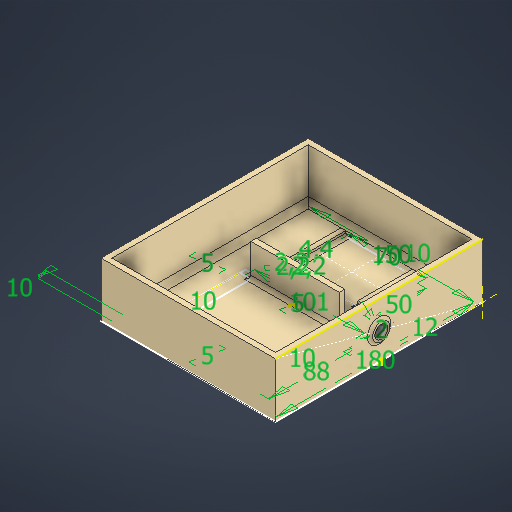
# Autodesk Inventor part: CaseBitDog
Saved by Autodesk Inventor 2027 (Build 310192000, 192)
## iProperties
Created: 2026-10-02
Part Number: CaseBitDog
Material: Genérico
Document SubType Name: Modeling
Designer: EspacoMaker
Density: 1 g/cm^3
Appearance: Padrão
Author: EspacoMaker
Autodesk Inventor part; units mm, degrees
ref_plane "YZ Plane" through (0, 0, 0) normal (1, 0, 0) x (0, 1, 0)
ref_plane "XZ Plane" through (0, 0, 0) normal (0, 1, 0) x (-1, 0, 0)
ref_plane "XY Plane" through (0, 0, 0) normal (0, 0, 1) x (1, 0, 0)
sketch "Esboço1" plane through (0, 0, 0) normal (0, 1, 0) x (-1, 0, 0)
  line L0 (75, 90) -> (-75, 90)
  line L1 (-75, 90) -> (-75, -90)
  line L2 (-75, -90) -> (75, -90)
  line L3 (75, -90) -> (75, 90)
  line L4 (75, 90) -> (-75, -90) construction
  line L5 (-75, 90) -> (75, -90) construction
  line L6 (50.5, 80) -> (-50.5, 80) construction
  line L7 (-50.5, 80) -> (-50.5, -8) construction
  line L8 (-50.5, -8) -> (50.5, -8) construction
  line L9 (50.5, -8) -> (50.5, 80) construction
  line L10 (50.5, 80) -> (-50.5, -8) construction
  line L11 (-50.5, 80) -> (50.5, -8) construction
  line L12 (35, -30) -> (-35, -30) construction
  line L13 (-35, -30) -> (-35, -80) construction
  line L14 (-35, -80) -> (35, -80) construction
  line L15 (35, -80) -> (35, -30) construction
  line L16 (35, -30) -> (-35, -80) construction
  line L17 (-35, -30) -> (35, -80) construction
  line L18 (0, 90) -> (0, -90) construction
  line L19 (80, 95) -> (-80, 95)
  line L20 (-80, 95) -> (-80, -95)
  line L21 (-80, -95) -> (80, -95)
  line L22 (80, -95) -> (80, 95)
  point P0 (0, 0)
  point P1 (0, 36)
  point P2 (0, -55)
  dimension "d0" = 150
  dimension "d1" = 180
  dimension "d2" = 101
  dimension "d3" = 88
  dimension "d4" = 70
  dimension "d5" = 50
  dimension "d6" = 10
  dimension "d7" = 10
  dimension "d8" = 5
  constraints: 46 end point, 8 midpoint, 8 parallel, 4 perpendicular, 3 horizontal, 2 point on line, 3 other
  measures "d0" distance of L2.end L1.end
  measures "d1" distance of L1.end L0.end
  measures "d2" distance of L8.end L7.end
  measures "d3" distance of L7.end L6.end
  measures "d4" distance of L14.end L13.end
  measures "d5" distance of L13.end L12.end
  measures "d6" distance between parallel lines of L2 L14
  measures "d7" distance between parallel lines of L0 L6
  measures "d8" distance between parallel lines of L3 L22
extrude "Extrusão1" add sketch "Esboço1" along normal blind 50
extrude "Extrusion2" add sketch "Esboço1" along normal blind 4 contours L3 L2 L1 L0
sketch "SaidaCarga" plane through (80, 0, 95) normal (1, 0, 0) x (0, 0, -1)
  line L0 (0, 50) -> (190, 50) projected
  line L1 (0, 50) -> (190, 0) construction
  circle A0 centre (95, 25) radius 6
  circle A1 centre (95, 25) radius 8
  point P0 (95, 0)
  dimension "d13" = 12
  dimension "d14" = 2
  constraints: 2 centre point, 2 end point, 1 midpoint
  measures "d13" diameter of A0
  measures "d14" radial gap between concentric circles of A0 A1
sketch "Sketch3" plane through (0, 4, 0) normal (0, 1, 0) x (1, 0, 0)
  line L0 (-50.5, -80) -> (50.5, -80) construction
  line L1 (50.5, -80) -> (50.5, 8) construction
  line L2 (-50.5, 8) -> (-50.5, -80) construction
  line L3 (50.5, 8) -> (-50.5, 8) construction
  line L4 (-35, 30) -> (35, 30) construction
  line L5 (35, 30) -> (35, 80) construction
  line L6 (35, 80) -> (-35, 80) construction
  line L7 (-35, 80) -> (-35, 30) construction
  line L8 (75, 90) -> (75, -90) projected
  line L9 (-75, 90) -> (75, 90) projected
  line L10 (-35, 30) -> (35, 30)
  line L11 (35, 30) -> (35, 80)
  line L12 (35, 80) -> (-35, 80)
  line L13 (-35, 80) -> (-35, 30)
  circle A0 centre (-32.8, 32.2) radius 1.1
  line L14 (-35, 55) -> (35, 55) construction
  circle A1 centre (-32.8, 77.8) radius 1.1
  line L15 (0, 30) -> (0, 80) construction
  circle A2 centre (32.8, 32.2) radius 1.1
  circle A3 centre (32.8, 77.8) radius 1.1
  line L16 (-30.6, 34.4) -> (-35, 30) construction
  line L17 (-35, 34.4) -> (-30.6, 30) construction
  line L18 (-30.6, 80) -> (-30.6, 30)
  line L19 (30.6, 80) -> (30.6, 30)
  line L20 (-50.5, -75) -> (50.5, -75)
  line L21 (-40.5, 8) -> (-40.5, -80)
  line L22 (50.5, 3) -> (-50.5, 3)
  line L23 (40.5, -80) -> (40.5, 8)
  line L24 (-50.5, 8) -> (50.5, 8)
  line L25 (50.5, 8) -> (50.5, -80)
  line L26 (50.5, -80) -> (-50.5, -80)
  line L27 (-50.5, -80) -> (-50.5, 8)
  point P0 (0, 0)
  point P1 (30.6, 30)
  point P2 (40.5, 8)
  point P3 (-40.5, 3)
  point P4 (40.5, 3)
  point P5 (40.5, -75)
  point P6 (-40.5, -75)
  dimension "d29" = 2.2
  dimension "d30" = 2.2
  dimension "d31" = 2.2
  dimension "d32" = 4.4
  dimension "d35" = 5
  dimension "d36" = 10
  dimension "d37" = 5
  dimension "d38" = 10
  constraints: 36 end point, 9 parallel, 6 midpoint, 5 symmetric about line, 4 centre point, 2 horizontal, 2 perpendicular, 3 other
  measures "d29" diameter of A0
  measures "d30" distance from line of A0.centre L4
  measures "d31" distance from line of L7 A0.centre
  measures "d32" distance between parallel lines of L13 L18
  measures "d35" distance between parallel lines of L0 L20
  measures "d36" distance between parallel lines of L2 L21
  measures "d37" distance between parallel lines of L3 L22
  measures "d38" distance between parallel lines of L1 L23
extrude "Extrusion5" cut sketch "SaidaCarga" against normal blind 5 contours A0
extrude "Extrusion6" add sketch "SaidaCarga" along normal blind 2 and the other way blind 7
extrude "Extrusion7" add sketch "Sketch3" along normal blind 5 contours L13 L12 L18 L10 | L19 L12 L11 L10 | A0 | A1 | A2 | A3
extrude "Extrusion8" add sketch "Sketch3" along normal blind 30 contours L20 L23 L26 L21 | L21 L24 L23 L22
fillet "Fillet1" radius 5 4 edges at (0, 4, -90) (-75, 4, 0) (0, 4, 90) (75, 4, 0)
fillet "Fillet2" radius 3 18 edges at (0, 4, -3) (40.5, 4, -5.5) (0, 4, -8) (-40.5, 4, -5.5) (0, 4, 75) (-40.5, 4, 77.5) (0, 4, 80) (40.5, 4, 77.5) (35, 4, -55) (30.6, 4, -55) (32.8, 4, -30) (32.8, 4, -80) (-30.6, 4, -55) (-32.8, 4, -30) (-35, 4, -55) (-32.8, 4, -80) (80, 25, 8) (75, 25, 8)
sketch "Esboço4" plane through (0, 4, 0) normal (0, 1, 0) x (1, 0, 0)
  line L0 (50.5, 8) -> (-50.5, 8) construction
  point P0 (0, 0)
